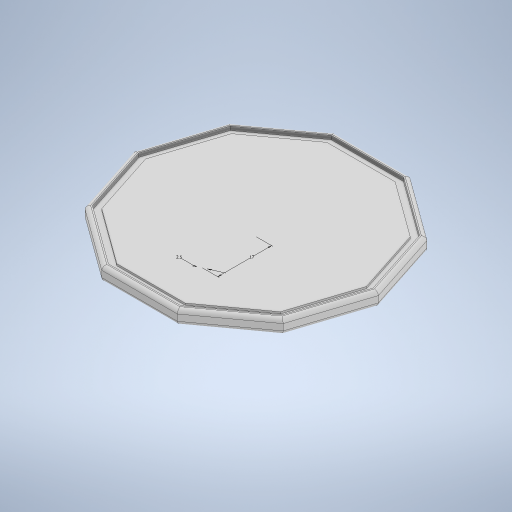
# Autodesk Inventor part: OV-PAM_n_10_bottom
Saved by Autodesk Inventor 2024 (Build 280153000, 153)
## iProperties
Created: 2023-08-31
Part Number: OV-PAM_n_10_bottom
Material: 일반
Document SubType Name: Modeling
Designer: jsw
Density: 1 g/cm^3
Appearance: 기본값
Author: jsw
Autodesk Inventor part; units mm, degrees
ref_plane "YZ Plane" through (0, 0, 0) normal (1, 0, 0) x (0, 1, 0)
ref_plane "XZ Plane" through (0, 0, 0) normal (0, 1, 0) x (-1, 0, 0)
ref_plane "XY Plane" through (0, 0, 0) normal (0, 0, 1) x (1, 0, 0)
sketch "스케치1" plane through (0, 0, 0) normal (0, 1, 0) x (-1, 0, 0)
  line L0 (-10.9012, 33.5504) -> (10.9012, 33.5504)
  line L1 (10.9012, 33.5504) -> (28.5397, 20.7353)
  line L2 (28.5397, 20.7353) -> (35.277, 0)
  line L3 (35.277, 0) -> (28.5397, -20.7353)
  line L4 (28.5397, -20.7353) -> (10.9012, -33.5504)
  line L5 (10.9012, -33.5504) -> (-10.9012, -33.5504)
  line L6 (-10.9012, -33.5504) -> (-28.5397, -20.7353)
  line L7 (-28.5397, -20.7353) -> (-35.277, 0)
  line L8 (-35.277, 0) -> (-28.5397, 20.7353)
  line L9 (-28.5397, 20.7353) -> (-10.9012, 33.5504)
  line L10 (11.9409, -36.7504) -> (-11.9409, -36.7504)
  line L11 (-11.9409, -36.7504) -> (-31.2618, -22.713)
  line L12 (-31.2618, -22.713) -> (-38.6417, 0)
  line L13 (-38.6417, 0) -> (-31.2618, 22.713)
  line L14 (-31.2618, 22.713) -> (-11.9409, 36.7504)
  line L15 (-11.9409, 36.7504) -> (11.9409, 36.7504)
  line L16 (11.9409, 36.7504) -> (31.2618, 22.713)
  line L17 (31.2618, 22.713) -> (38.6417, 0)
  line L18 (38.6417, 0) -> (31.2618, -22.713)
  line L19 (31.2618, -22.713) -> (11.9409, -36.7504)
  point P0 (0, 0)
  point P1 (0, 0)
  point P2 (0, 0)
  dimension "d0" = 70.554
  dimension "d1" = 3.2
  constraints: 40 end point, 2 coincident, 2 horizontal, 42 other
  measures "d0" distance of L7.end L2.end
  measures "d1" distance between parallel lines of L3 L18
extrude "돌출1" add sketch "스케치1" along normal blind 4.4 contours L0 L1 L2 L3 L4 L5 L6 L7 L8 L9 | L10 L11 L12 L13 L14 L15 L16 L17 L18 L19
sketch "스케치2" plane through (0, 4.4, 0) normal (0, 1, 0) x (1, 0, 0)
  line L0 (-11.4211, 35.1504) -> (11.4211, 35.1504)
  line L1 (11.4211, 35.1504) -> (29.9007, 21.7242)
  line L2 (29.9007, 21.7242) -> (36.9593, 0)
  line L3 (36.9593, 0) -> (29.9007, -21.7242)
  line L4 (29.9007, -21.7242) -> (11.4211, -35.1504)
  line L5 (11.4211, -35.1504) -> (-11.4211, -35.1504)
  line L6 (-11.4211, -35.1504) -> (-29.9007, -21.7242)
  line L7 (-29.9007, -21.7242) -> (-36.9593, 0)
  line L8 (-36.9593, 0) -> (-29.9007, 21.7242)
  line L9 (-29.9007, 21.7242) -> (-11.4211, 35.1504)
  line L10 (-31.2618, 22.713) -> (-38.6417, 0) projected
  point P0 (0, 0)
  point P1 (0, 0)
  dimension "d4" = 1.6
  constraints: 20 end point, 1 coincident, 1 horizontal, 21 other
  measures "d4" distance between parallel lines of L8 L10
extrude "돌출2" cut sketch "스케치2" against normal blind 1.2
sketch "스케치3" plane through (0, 3.2, 0) normal (0, 1, 0) x (1, 0, 0)
  line L0 (-10.7712, 33.1504) -> (10.7712, 33.1504)
  line L1 (10.7712, 33.1504) -> (28.1994, 20.4881)
  line L2 (28.1994, 20.4881) -> (34.8564, 0)
  line L3 (34.8564, 0) -> (28.1994, -20.4881)
  line L4 (28.1994, -20.4881) -> (10.7712, -33.1504)
  line L5 (10.7712, -33.1504) -> (-10.7712, -33.1504)
  line L6 (-10.7712, -33.1504) -> (-28.1994, -20.4881)
  line L7 (-28.1994, -20.4881) -> (-34.8564, 0)
  line L8 (-34.8564, 0) -> (-28.1994, 20.4881)
  line L9 (-28.1994, 20.4881) -> (-10.7712, 33.1504)
  line L10 (-29.9007, 21.7242) -> (-11.4211, 35.1504) projected
  point P0 (0, 0)
  point P1 (0, 0)
  dimension "d7" = 2
  constraints: 20 end point, 1 coincident, 1 horizontal, 21 other
  measures "d7" distance between parallel lines of L10 L9
extrude "돌출3" add sketch "스케치3" along normal blind 0.6
fillet "모깎기1" radius 1.2 20 edges at (0, 4.4, 36.7504) (0, 0, 36.7504) (-21.6014, 4.4, 29.7317) (-21.6014, 0, 29.7317) (-34.9517, 4.4, 11.3565) (-34.9517, 4.4, -11.3565) (-21.6014, 4.4, -29.7317) (0, 4.4, -36.7504) (21.6014, 4.4, -29.7317) (34.9517, 4.4, -11.3565) (34.9517, 4.4, 11.3565) (21.6014, 4.4, 29.7317) (21.6014, 0, -29.7317) (0, 0, -36.7504) (-21.6014, 0, -29.7317) (-34.9517, 0, -11.3565) (-34.9517, 0, 11.3565) (34.9517, 0, -11.3565) (34.9517, 0, 11.3565) (21.6014, 0, 29.7317)
sketch "스케치6" plane through (0, 0, 0) normal (0, -1, 0) x (1, 0, 0)
  line L0 (-20, -2.5) -> (-10, -2.5)
  line L1 (-10, -2.5) -> (-10, 2.5)
  line L2 (-10, 2.5) -> (-20, 2.5)
  line L3 (-20, 2.5) -> (-20, -2.5)
  line L4 (-20, -2.5) -> (-10, 2.5) construction
  line L5 (-10, -2.5) -> (-20, 2.5) construction
  line L6 (10, -2.5) -> (20, -2.5)
  line L7 (20, -2.5) -> (20, 2.5)
  line L8 (20, 2.5) -> (10, 2.5)
  line L9 (10, 2.5) -> (10, -2.5)
  line L10 (10, -2.5) -> (20, 2.5) construction
  line L11 (20, -2.5) -> (10, 2.5) construction
  point P0 (0, 0)
  point P1 (-15, 0)
  point P2 (15, 0)
  dimension "d26" = 10
  dimension "d27" = 5
  dimension "d28" = 10
  dimension "d29" = 5
  dimension "d30" = 20
  dimension "d31" = 10
  constraints: 24 end point, 4 midpoint, 4 parallel, 2 horizontal, 2 horizontal alignment, 2 perpendicular
  measures "d26" distance of L2.end L1.end
  measures "d27" distance of L1.end L0.end
  measures "d28" distance of L8.end L7.end
  measures "d29" distance of L7.end L6.end
  measures "d30" distance between parallel lines of L1 L9
  measures "d31" distance from line of L1 point (0, 0)
extrude "돌출6" add sketch "스케치6" along normal blind 10
sketch "스케치7" plane through (-20, 0, 2.5) normal (0, 0, 1) x (1, 0, 0)
  line L0 (10, -10) -> (0, -10) projected
  circle A0 centre (5, -10) radius 5
  line L1 (40, -10) -> (30, -10) projected
  circle A1 centre (35, -10) radius 5
  point P0 (20, 0)
  constraints: 2 horizontal alignment, 2 midpoint, 4 other
extrude "돌출7" add sketch "스케치7" against normal blind 5
sketch "스케치8" plane through (10, 0, 2.5) normal (0, 0, 1) x (1, 0, 0)
  arc A0 (0, -10) -> (10, -10) centre (5, -10) ccw projected
  circle A1 centre (5, -10) radius 1.25
  arc A2 (-30, -10) -> (-20, -10) centre (-25, -10) ccw projected
  circle A3 centre (-25, -10) radius 1.25
  point P0 (-10, 0)
  dimension "d36" = 2.5
  dimension "d37" = 2.5
  constraints: 2 centre point, 2 coincident
  measures "d36" diameter of A1
  measures "d37" diameter of A3
extrude "돌출8" cut sketch "스케치8" against normal blind 5
sketch "스케치10" plane through (0, 0, 0) normal (0, -1, 0) x (1, 0, 0)
  line L0 (-10, -2.5) -> (-20, -2.5) projected
  line L1 (-20, 2.5) -> (-10, 2.5) projected
  line L2 (-20, -2.5) -> (-19, -2.5)
  line L3 (-19, -2.5) -> (-19, 2.5)
  line L4 (-19, 2.5) -> (-20, 2.5)
  line L5 (-20, 2.5) -> (-20, -2.5)
  line L6 (20, -2.5) -> (20, 2.5) projected
  line L7 (20, -2.5) -> (10, -2.5) projected
  line L8 (20, 2.5) -> (19, 2.5)
  line L9 (19, 2.5) -> (19, -2.5)
  line L10 (19, -2.5) -> (20, -2.5)
  line L11 (20, -2.5) -> (20, 2.5)
  point P0 (0, 0)
  dimension "d45" = 1
  dimension "d46" = 1
  constraints: 16 end point, 4 parallel, 2 horizontal, 2 perpendicular, 2 point on line
  measures "d45" distance of L4.end L3.end
  measures "d46" distance of L10.end L9.end
extrude "돌출10" cut sketch "스케치10" along normal blind 15
sketch "스케치11" plane through (0, 0, 0) normal (0, -1, 0) x (1, 0, 0)
  circle A0 centre (0, 17) radius 1.25
  point P0 (0, 0)
  dimension "d49" = 2.5
  dimension "d50" = 17
  constraints: 1 centre point, 1 vertical alignment
  measures "d49" diameter of A0
  measures "d50" distance of point (0, 0) A0.centre
equation "\"d31\" = 0.5 * d30"
